Autodesk Inventor part; units mm, degrees
(part 3 of 7)
  arc A347 (-153.3618, 85.9364) -> (-153.2072, 86.2055) centre (-157.8537, 88.696) ccw projected
  arc A348 (-153.5785, 85.6068) -> (-153.3618, 85.9364) centre (-158.8215, 89.2905) ccw projected
  arc A349 (-153.872, 85.2164) -> (-153.5785, 85.6068) centre (-159.7867, 89.9687) ccw projected
  arc A350 (-154.2565, 85.3248) -> (-153.872, 85.2164) centre (-148.5, 105) ccw projected
  arc A351 (-154.3028, 85.8111) -> (-154.2565, 85.3248) centre (-146.7304, 86.2864) ccw projected
  arc A352 (-154.3154, 86.2053) -> (-154.3028, 85.8111) centre (-147.9076, 86.2125) ccw projected
  arc A353 (-154.3066, 86.5156) -> (-154.3154, 86.2053) centre (-149.0434, 86.2112) ccw projected
  arc A354 (-154.6673, 86.6328) -> (-154.3066, 86.5156) centre (-148.5, 105) ccw projected
  arc A355 (-154.8425, 86.3766) -> (-154.6673, 86.6328) centre (-159.1041, 89.4801) ccw projected
  arc A356 (-155.0844, 86.0651) -> (-154.8425, 86.3766) centre (-160.0222, 90.1488) ccw projected
  arc A357 (-155.4077, 85.6989) -> (-155.0844, 86.0651) centre (-160.9312, 90.9006) ccw projected
  arc A358 (-155.7825, 85.8371) -> (-155.4077, 85.6989) centre (-148.5, 105) ccw projected
  arc A359 (-155.7904, 86.3255) -> (-155.7825, 85.8371) centre (-148.2041, 86.2053) ccw projected
  arc A360 (-155.772, 86.7195) -> (-155.7904, 86.3255) centre (-149.3835, 86.224) ccw projected
  arc A361 (-155.7389, 87.0281) -> (-155.772, 86.7195) centre (-150.5159, 86.3118) ccw projected
  arc A362 (-156.0893, 87.1733) -> (-155.7389, 87.0281) centre (-148.5, 105) ccw projected
  arc A363 (-156.2842, 86.9316) -> (-156.0893, 87.1733) centre (-160.2891, 90.36) ccw projected
  arc A364 (-156.5497, 86.64) -> (-156.2842, 86.9316) centre (-161.1519, 91.0986) ccw projected
  arc A365 (-156.9007, 86.3003) -> (-156.5497, 86.64) centre (-161.9991, 91.9194) ccw projected
  arc A366 (-157.2635, 86.4676) -> (-156.9007, 86.3003) centre (-148.5, 105) ccw projected
  arc A367 (-157.2331, 86.9551) -> (-157.2635, 86.4676) centre (-149.6796, 86.24) ccw projected
  arc A368 (-157.1839, 87.3464) -> (-157.2331, 86.9551) centre (-150.8539, 86.3512) ccw projected
  arc A369 (-157.1267, 87.6515) -> (-157.1839, 87.3464) centre (-151.976, 86.5276) ccw projected
  arc A370 (-157.4646, 87.8237) -> (-157.1267, 87.6515) centre (-148.5, 105) ccw projected
  arc A371 (-157.6778, 87.5981) -> (-157.4646, 87.8237) centre (-161.4014, 91.3301) ccw projected
  arc A372 (-157.9654, 87.3282) -> (-157.6778, 87.5981) centre (-162.2036, 92.1341) ccw projected
  arc A373 (-158.342, 87.0171) -> (-157.9654, 87.3282) centre (-162.9838, 93.0188) ccw projected
  arc A374 (-158.6905, 87.2123) -> (-158.342, 87.0171) centre (-148.5, 105) ccw projected
  arc A375 (-158.622, 87.6959) -> (-158.6905, 87.2123) centre (-151.1478, 86.3904) ccw projected
  arc A376 (-158.5422, 88.0822) -> (-158.622, 87.6959) centre (-152.3099, 86.5933) ccw projected
  arc A377 (-158.4612, 88.3818) -> (-158.5422, 88.0822) centre (-153.4146, 86.8572) ccw projected
  arc A378 (-158.7846, 88.58) -> (-158.4612, 88.3818) centre (-148.5, 105) ccw projected
  arc A379 (-159.0148, 88.3718) -> (-158.7846, 88.58) centre (-162.4341, 92.3844) ccw projected
  arc A380 (-159.3227, 88.1253) -> (-159.0148, 88.3718) centre (-163.1708, 93.2489) ccw projected
  arc A381 (-159.7226, 87.8447) -> (-159.3227, 88.1253) centre (-163.8792, 94.1922) ccw projected
  arc A382 (-160.0547, 88.0666) -> (-159.7226, 87.8447) centre (-148.5, 105) ccw projected
  arc A383 (-159.9485, 88.5434) -> (-160.0547, 88.0666) centre (-152.5998, 86.6555) ccw projected
  arc A384 (-159.8386, 88.9222) -> (-159.9485, 88.5434) centre (-153.7423, 86.949) ccw projected
  arc A385 (-159.7344, 89.2146) -> (-159.8386, 88.9222) centre (-154.8229, 87.2988) ccw projected
  arc A386 (-160.0412, 89.4375) -> (-159.7344, 89.2146) centre (-148.5, 105) ccw projected
  arc A387 (-160.2871, 89.248) -> (-160.0412, 89.4375) centre (-163.381, 93.5166) ccw projected
  arc A388 (-160.6134, 89.0265) -> (-160.2871, 89.248) centre (-164.0476, 94.4362) ccw projected
  arc A389 (-161.034, 88.7781) -> (-160.6134, 89.0265) centre (-164.6798, 95.4321) ccw projected
  arc A390 (-161.3477, 89.0254) -> (-161.034, 88.7781) centre (-148.5, 105) ccw projected
  arc A391 (-161.2043, 89.4924) -> (-161.3477, 89.0254) centre (-154.0264, 87.0337) ccw projected
  arc A392 (-161.0651, 89.8614) -> (-161.2043, 89.4924) centre (-155.1424, 87.4159) ccw projected
  arc A393 (-160.9383, 90.1447) -> (-161.0651, 89.8614) centre (-156.1922, 87.8494) ccw projected
  arc A394 (-161.2266, 90.391) -> (-160.9383, 90.1447) centre (-148.5, 105) ccw projected
  arc A395 (-161.4866, 90.2214) -> (-161.2266, 90.391) centre (-164.2361, 94.7195) ccw projected
  arc A396 (-161.8293, 90.0261) -> (-161.4866, 90.2214) centre (-164.8285, 95.6886) ccw projected
  arc A397 (-162.2681, 89.8115) -> (-161.8293, 90.0261) centre (-165.3806, 96.7311) ccw projected
  arc A398 (-162.5614, 90.0827) -> (-162.2681, 89.8115) centre (-148.5, 105) ccw projected
  arc A399 (-162.3819, 90.537) -> (-162.5614, 90.0827) centre (-155.419, 87.5227) ccw projected
  arc A400 (-162.2141, 90.8939) -> (-162.3819, 90.537) centre (-156.5015, 87.9913) ccw projected
  arc A401 (-162.0655, 91.1664) -> (-162.2141, 90.8939) centre (-157.5141, 88.5058) ccw projected
  arc A402 (-162.3336, 91.4345) -> (-162.0655, 91.1664) centre (-148.5, 105) ccw projected
  arc A403 (-162.6061, 91.2859) -> (-162.3336, 91.4345) centre (-164.9942, 95.9859) ccw projected
  arc A404 (-162.963, 91.1181) -> (-162.6061, 91.2859) centre (-165.5087, 96.9985) ccw projected
  arc A405 (-163.4173, 90.9386) -> (-162.963, 91.1181) centre (-165.9773, 98.081) ccw projected
  arc A406 (-163.6885, 91.2319) -> (-163.4173, 90.9386) centre (-148.5, 105) ccw projected
  arc A407 (-163.4738, 91.6707) -> (-163.6885, 91.2319) centre (-156.7689, 88.1194) ccw projected
  arc A408 (-163.2786, 92.0134) -> (-163.4738, 91.6707) centre (-157.8114, 88.6715) ccw projected
  arc A409 (-163.109, 92.2734) -> (-163.2786, 92.0134) centre (-158.7805, 89.2639) ccw projected
  arc A410 (-163.3553, 92.5617) -> (-163.109, 92.2734) centre (-148.5, 105) ccw projected
  arc A411 (-163.6386, 92.4349) -> (-163.3553, 92.5617) centre (-165.6506, 97.3078) ccw projected
  arc A412 (-164.0076, 92.2957) -> (-163.6386, 92.4349) centre (-166.0841, 98.3576) ccw projected
  arc A413 (-164.4746, 92.1523) -> (-164.0076, 92.2957) centre (-166.4663, 99.4736) ccw projected
  arc A414 (-164.7219, 92.466) -> (-164.4746, 92.1523) centre (-148.5, 105) ccw projected
  arc A415 (-164.4735, 92.8866) -> (-164.7219, 92.466) centre (-158.0679, 88.8202) ccw projected
  arc A416 (-164.252, 93.2129) -> (-164.4735, 92.8866) centre (-159.0638, 89.4524) ccw projected
  arc A417 (-164.0625, 93.4588) -> (-164.252, 93.2129) centre (-159.9834, 90.119) ccw projected
  arc A418 (-164.2854, 93.7656) -> (-164.0625, 93.4588) centre (-148.5, 105) ccw projected
  arc A419 (-164.5778, 93.6614) -> (-164.2854, 93.7656) centre (-166.2012, 98.6771) ccw projected
  arc A420 (-164.9566, 93.5515) -> (-164.5778, 93.6614) centre (-166.551, 99.7577) ccw projected
  arc A421 (-165.4334, 93.4453) -> (-164.9566, 93.5515) centre (-166.8445, 100.9002) ccw projected
  arc A422 (-165.6553, 93.7774) -> (-165.4334, 93.4453) centre (-148.5, 105) ccw projected
  arc A423 (-165.3747, 94.1773) -> (-165.6553, 93.7774) centre (-159.3078, 89.6208) ccw projected
  arc A424 (-165.1282, 94.4852) -> (-165.3747, 94.1773) centre (-160.2511, 90.3292) ccw projected
  arc A425 (-164.92, 94.7154) -> (-165.1282, 94.4852) centre (-161.1156, 91.0659) ccw projected
  arc A426 (-165.1182, 95.0388) -> (-164.92, 94.7154) centre (-148.5, 105) ccw projected
  arc A427 (-165.4178, 94.9578) -> (-165.1182, 95.0388) centre (-166.6428, 100.0854) ccw projected
  arc A428 (-165.8041, 94.878) -> (-165.4178, 94.9578) centre (-166.9067, 101.1901) ccw projected
  arc A429 (-166.2877, 94.8095) -> (-165.8041, 94.878) centre (-167.1096, 102.3522) ccw projected
  arc A430 (-166.4829, 95.158) -> (-166.2877, 94.8095) centre (-148.5, 105) ccw projected
  arc A431 (-166.1718, 95.5346) -> (-166.4829, 95.158) centre (-160.4812, 90.5162) ccw projected
  arc A432 (-165.9019, 95.8222) -> (-166.1718, 95.5346) centre (-161.3659, 91.2964) ccw projected
  arc A433 (-165.6763, 96.0354) -> (-165.9019, 95.8222) centre (-162.1699, 92.0986) ccw projected
  arc A434 (-165.8485, 96.3733) -> (-165.6763, 96.0354) centre (-148.5, 105) ccw projected
  arc A435 (-166.1536, 96.3161) -> (-165.8485, 96.3733) centre (-166.9724, 101.524) ccw projected
  arc A436 (-166.5449, 96.2669) -> (-166.1536, 96.3161) centre (-167.1488, 102.6461) ccw projected
  arc A437 (-167.0324, 96.2365) -> (-166.5449, 96.2669) centre (-167.26, 103.8204) ccw projected
  arc A438 (-167.1997, 96.5993) -> (-167.0324, 96.2365) centre (-148.5, 105) ccw projected
  arc A439 (-166.86, 96.9503) -> (-167.1997, 96.5993) centre (-161.5806, 91.5009) ccw projected
  arc A440 (-166.5684, 97.2158) -> (-166.86, 96.9503) centre (-162.4014, 92.3481) ccw projected
  arc A441 (-166.3267, 97.4107) -> (-166.5684, 97.2158) centre (-163.14, 93.2109) ccw projected
  arc A442 (-166.4719, 97.7611) -> (-166.3267, 97.4107) centre (-148.5, 105) ccw projected
  arc A443 (-166.7805, 97.728) -> (-166.4719, 97.7611) centre (-167.1882, 102.9841) ccw projected
  arc A444 (-167.1745, 97.7096) -> (-166.7805, 97.728) centre (-167.276, 104.1165) ccw projected
  arc A445 (-167.6629, 97.7175) -> (-167.1745, 97.7096) centre (-167.2947, 105.2959) ccw projected
  arc A446 (-167.8011, 98.0923) -> (-167.6629, 97.7175) centre (-148.5, 105) ccw projected
  arc A447 (-167.4349, 98.4156) -> (-167.8011, 98.0923) centre (-162.5994, 92.5688) ccw projected
  arc A448 (-167.1234, 98.6575) -> (-167.4349, 98.4156) centre (-163.3512, 93.4778) ccw projected
  arc A449 (-166.8672, 98.8327) -> (-167.1234, 98.6575) centre (-164.0199, 94.3959) ccw projected
  arc A450 (-166.9844, 99.1934) -> (-166.8672, 98.8327) centre (-148.5, 105) ccw projected
  arc A451 (-167.2947, 99.1846) -> (-166.9844, 99.1934) centre (-167.2888, 104.4566) ccw projected
  arc A452 (-167.6889, 99.1972) -> (-167.2947, 99.1846) centre (-167.2875, 105.5924) ccw projected
  arc A453 (-168.1752, 99.2435) -> (-167.6889, 99.1972) centre (-167.2136, 106.7696) ccw projected
  arc A454 (-168.2836, 99.628) -> (-168.1752, 99.2435) centre (-148.5, 105) ccw projected
  arc A455 (-167.8932, 99.9215) -> (-168.2836, 99.628) centre (-163.5313, 93.7133) ccw projected
  arc A456 (-167.5636, 100.1382) -> (-167.8932, 99.9215) centre (-164.2095, 94.6785) ccw projected
  arc A457 (-167.2945, 100.2928) -> (-167.5636, 100.1382) centre (-164.804, 95.6463) ccw projected
  arc A458 (-167.383, 100.6616) -> (-167.2945, 100.2928) centre (-148.5, 105) ccw projected
  arc A459 (-167.693, 100.6772) -> (-167.383, 100.6616) centre (-167.2735, 105.9324) ccw projected
  arc A460 (-168.085, 100.7207) -> (-167.693, 100.6772) centre (-167.1831, 107.0646) ccw projected
  arc A461 (-168.5662, 100.8049) -> (-168.085, 100.7207) centre (-167.017, 108.2324) ccw projected
  arc A462 (-168.6441, 101.1967) -> (-168.5662, 100.8049) centre (-148.5, 105) ccw projected
  arc A463 (-168.2318, 101.4587) -> (-168.6441, 101.1967) centre (-164.3705, 94.9274) ccw projected
  arc A464 (-167.8863, 101.6489) -> (-168.2318, 101.4587) centre (-164.9708, 95.9429) ccw projected
  arc A465 (-167.6059, 101.7819) -> (-167.8863, 101.6489) centre (-165.4876, 96.9543) ccw projected
  arc A466 (-167.6652, 102.1565) -> (-167.6059, 101.7819) centre (-148.5, 105) ccw projected
  arc A467 (-167.973, 102.1964) -> (-167.6652, 102.1565) centre (-167.1425, 107.4025) ccw projected
  arc A468 (-168.3604, 102.2705) -> (-167.973, 102.1964) centre (-166.9635, 108.5241) ccw projected
  arc A469 (-168.8335, 102.3922) -> (-168.3604, 102.2705) centre (-166.7064, 109.6753) ccw projected
  arc A470 (-168.8804, 102.7889) -> (-168.8335, 102.3922) centre (-148.5, 105) ccw projected
  arc A471 (-168.4489, 103.0178) -> (-168.8804, 102.7889) centre (-165.1119, 96.2037) ccw projected
  arc A472 (-168.0895, 103.1803) -> (-168.4489, 103.0178) centre (-165.6307, 97.2631) ccw projected
  arc A473 (-167.7995, 103.2909) -> (-168.0895, 103.1803) centre (-166.0665, 98.3119) ccw projected
  arc A474 (-167.8292, 103.669) -> (-167.7995, 103.2909) centre (-148.5, 105) ccw projected
  arc A475 (-168.133, 103.7329) -> (-167.8292, 103.669) centre (-166.8965, 108.8577) ccw projected
  arc A476 (-168.5133, 103.8371) -> (-168.133, 103.7329) centre (-166.6301, 109.9618) ccw projected
  arc A477 (-168.9754, 103.9956) -> (-168.5133, 103.8371) centre (-166.2834, 111.0894) ccw projected
  arc A478 (-168.9911, 104.3948) -> (-168.9754, 103.9956) centre (-148.5, 105) ccw projected
  arc A479 (-168.5429, 104.5891) -> (-168.9911, 104.3948) centre (-165.7508, 97.5342) ccw projected
  arc A480 (-168.1719, 104.7229) -> (-168.5429, 104.5891) centre (-166.1849, 98.631) ccw projected
  arc A481 (-167.8741, 104.8104) -> (-168.1719, 104.7229) centre (-166.5371, 99.7108) ccw projected
  arc A482 (-167.8741, 105.1896) -> (-167.8741, 104.8104) centre (-148.5, 105) ccw projected
  arc A483 (-168.1719, 105.2771) -> (-167.8741, 105.1896) centre (-166.5371, 110.2892) ccw projected
  arc A484 (-168.5429, 105.4109) -> (-168.1719, 105.2771) centre (-166.1849, 111.369) ccw projected
  arc A485 (-168.9911, 105.6052) -> (-168.5429, 105.4109) centre (-165.7508, 112.4658) ccw projected
  arc A486 (-168.9754, 106.0044) -> (-168.9911, 105.6052) centre (-148.5, 105) ccw projected
  arc A487 (-168.5133, 106.1629) -> (-168.9754, 106.0044) centre (-166.2834, 98.9106) ccw projected
  arc A488 (-168.133, 106.2671) -> (-168.5133, 106.1629) centre (-166.6301, 100.0382) ccw projected
  arc A489 (-167.8292, 106.331) -> (-168.133, 106.2671) centre (-166.8965, 101.1423) ccw projected
  arc A490 (-167.7995, 106.7091) -> (-167.8292, 106.331) centre (-148.5, 105) ccw projected
  arc A491 (-168.0895, 106.8197) -> (-167.7995, 106.7091) centre (-166.0665, 111.6881) ccw projected
  arc A492 (-168.4489, 106.9822) -> (-168.0895, 106.8197) centre (-165.6307, 112.7369) ccw projected
  arc A493 (-168.8804, 107.2111) -> (-168.4489, 106.9822) centre (-165.1119, 113.7963) ccw projected
  arc A494 (-168.8335, 107.6078) -> (-168.8804, 107.2111) centre (-148.5, 105) ccw projected
  arc A495 (-168.3604, 107.7295) -> (-168.8335, 107.6078) centre (-166.7064, 100.3247) ccw projected
  arc A496 (-167.973, 107.8036) -> (-168.3604, 107.7295) centre (-166.9635, 101.4759) ccw projected
  arc A497 (-167.6652, 107.8435) -> (-167.973, 107.8036) centre (-167.1425, 102.5975) ccw projected
  arc A498 (-167.6059, 108.2181) -> (-167.6652, 107.8435) centre (-148.5, 105) ccw projected
  arc A499 (-167.8863, 108.3511) -> (-167.6059, 108.2181) centre (-165.4876, 113.0457) ccw projected
  arc A500 (-168.2318, 108.5413) -> (-167.8863, 108.3511) centre (-164.9708, 114.0571) ccw projected
  arc A501 (-168.6441, 108.8033) -> (-168.2318, 108.5413) centre (-164.3705, 115.0726) ccw projected
  arc A502 (-168.5662, 109.1951) -> (-168.6441, 108.8033) centre (-148.5, 105) ccw projected
  arc A503 (-168.085, 109.2793) -> (-168.5662, 109.1951) centre (-167.017, 101.7676) ccw projected
  arc A504 (-167.693, 109.3228) -> (-168.085, 109.2793) centre (-167.1831, 102.9354) ccw projected
  arc A505 (-167.383, 109.3384) -> (-167.693, 109.3228) centre (-167.2735, 104.0676) ccw projected
  arc A506 (-167.2945, 109.7072) -> (-167.383, 109.3384) centre (-148.5, 105) ccw projected
  arc A507 (-167.5636, 109.8618) -> (-167.2945, 109.7072) centre (-164.804, 114.3537) ccw projected
  arc A508 (-167.8932, 110.0785) -> (-167.5636, 109.8618) centre (-164.2095, 115.3215) ccw projected
  arc A509 (-168.2836, 110.372) -> (-167.8932, 110.0785) centre (-163.5313, 116.2867) ccw projected
  arc A510 (-168.1752, 110.7565) -> (-168.2836, 110.372) centre (-148.5, 105) ccw projected
  arc A511 (-167.6889, 110.8028) -> (-168.1752, 110.7565) centre (-167.2136, 103.2304) ccw projected
  arc A512 (-167.2947, 110.8154) -> (-167.6889, 110.8028) centre (-167.2875, 104.4076) ccw projected
  arc A513 (-166.9844, 110.8066) -> (-167.2947, 110.8154) centre (-167.2888, 105.5434) ccw projected
  arc A514 (-166.8672, 111.1673) -> (-166.9844, 110.8066) centre (-148.5, 105) ccw projected
  arc A515 (-167.1234, 111.3425) -> (-166.8672, 111.1673) centre (-164.0199, 115.6041) ccw projected
  arc A516 (-167.4349, 111.5844) -> (-167.1234, 111.3425) centre (-163.3512, 116.5222) ccw projected
  arc A517 (-167.8011, 111.9077) -> (-167.4349, 111.5844) centre (-162.5994, 117.4312) ccw projected
  arc A518 (-167.6629, 112.2825) -> (-167.8011, 111.9077) centre (-148.5, 105) ccw projected
  arc A519 (-167.1745, 112.2904) -> (-167.6629, 112.2825) centre (-167.2947, 104.7041) ccw projected
  arc A520 (-166.7805, 112.272) -> (-167.1745, 112.2904) centre (-167.276, 105.8835) ccw projected
  arc A521 (-166.4719, 112.2389) -> (-166.7805, 112.272) centre (-167.1882, 107.0159) ccw projected
  arc A522 (-166.3267, 112.5893) -> (-166.4719, 112.2389) centre (-148.5, 105) ccw projected
  arc A523 (-166.5684, 112.7842) -> (-166.3267, 112.5893) centre (-163.14, 116.7891) ccw projected
  arc A524 (-166.86, 113.0497) -> (-166.5684, 112.7842) centre (-162.4014, 117.6519) ccw projected
  arc A525 (-167.1997, 113.4007) -> (-166.86, 113.0497) centre (-161.5806, 118.4991) ccw projected
  arc A526 (-167.0324, 113.7635) -> (-167.1997, 113.4007) centre (-148.5, 105) ccw projected
  arc A527 (-166.5449, 113.7331) -> (-167.0324, 113.7635) centre (-167.26, 106.1796) ccw projected
  arc A528 (-166.1536, 113.6839) -> (-166.5449, 113.7331) centre (-167.1488, 107.3539) ccw projected
  arc A529 (-165.8485, 113.6267) -> (-166.1536, 113.6839) centre (-166.9724, 108.476) ccw projected
  arc A530 (-165.6763, 113.9646) -> (-165.8485, 113.6267) centre (-148.5, 105) ccw projected
  arc A531 (-165.9019, 114.1778) -> (-165.6763, 113.9646) centre (-162.1699, 117.9014) ccw projected
  arc A532 (-166.1718, 114.4654) -> (-165.9019, 114.1778) centre (-161.3659, 118.7036) ccw projected
  arc A533 (-166.4829, 114.842) -> (-166.1718, 114.4654) centre (-160.4812, 119.4838) ccw projected
  arc A534 (-166.2877, 115.1905) -> (-166.4829, 114.842) centre (-148.5, 105) ccw projected
  arc A535 (-165.8041, 115.122) -> (-166.2877, 115.1905) centre (-167.1096, 107.6478) ccw projected
  arc A536 (-165.4178, 115.0422) -> (-165.8041, 115.122) centre (-166.9067, 108.8099) ccw projected
  arc A537 (-165.1182, 114.9612) -> (-165.4178, 115.0422) centre (-166.6428, 109.9146) ccw projected
  arc A538 (-164.92, 115.2846) -> (-165.1182, 114.9612) centre (-148.5, 105) ccw projected
  arc A539 (-165.1282, 115.5148) -> (-164.92, 115.2846) centre (-161.1156, 118.9341) ccw projected
  arc A540 (-165.3747, 115.8227) -> (-165.1282, 115.5148) centre (-160.2511, 119.6708) ccw projected
  arc A541 (-165.6553, 116.2226) -> (-165.3747, 115.8227) centre (-159.3078, 120.3792) ccw projected
  arc A542 (-165.4334, 116.5547) -> (-165.6553, 116.2226) centre (-148.5, 105) ccw projected
  arc A543 (-164.9566, 116.4485) -> (-165.4334, 116.5547) centre (-166.8445, 109.0998) ccw projected
  arc A544 (-164.5778, 116.3386) -> (-164.9566, 116.4485) centre (-166.551, 110.2423) ccw projected
  arc A545 (-164.2854, 116.2344) -> (-164.5778, 116.3386) centre (-166.2012, 111.3229) ccw projected
  arc A546 (-164.0625, 116.5412) -> (-164.2854, 116.2344) centre (-148.5, 105) ccw projected
  arc A547 (-164.252, 116.7871) -> (-164.0625, 116.5412) centre (-159.9834, 119.881) ccw projected
  arc A548 (-164.4735, 117.1134) -> (-164.252, 116.7871) centre (-159.0638, 120.5476) ccw projected
  arc A549 (-164.7219, 117.534) -> (-164.4735, 117.1134) centre (-158.0679, 121.1798) ccw projected
  arc A550 (-164.4746, 117.8477) -> (-164.7219, 117.534) centre (-148.5, 105) ccw projected
  arc A551 (-164.0076, 117.7043) -> (-164.4746, 117.8477) centre (-166.4663, 110.5264) ccw projected
  arc A552 (-163.6386, 117.5651) -> (-164.0076, 117.7043) centre (-166.0841, 111.6424) ccw projected
  arc A553 (-163.3553, 117.4383) -> (-163.6386, 117.5651) centre (-165.6506, 112.6922) ccw projected
  arc A554 (-163.109, 117.7266) -> (-163.3553, 117.4383) centre (-148.5, 105) ccw projected
  arc A555 (-163.2786, 117.9866) -> (-163.109, 117.7266) centre (-158.7805, 120.7361) ccw projected
  arc A556 (-163.4738, 118.3293) -> (-163.2786, 117.9866) centre (-157.8114, 121.3285) ccw projected
  arc A557 (-163.6885, 118.7681) -> (-163.4738, 118.3293) centre (-156.7689, 121.8806) ccw projected
  arc A558 (-163.4173, 119.0614) -> (-163.6885, 118.7681) centre (-148.5, 105) ccw projected
  arc A559 (-162.963, 118.8819) -> (-163.4173, 119.0614) centre (-165.9773, 111.919) ccw projected
  arc A560 (-162.6061, 118.7141) -> (-162.963, 118.8819) centre (-165.5087, 113.0015) ccw projected
  arc A561 (-162.3336, 118.5655) -> (-162.6061, 118.7141) centre (-164.9942, 114.0141) ccw projected
  arc A562 (-162.0655, 118.8336) -> (-162.3336, 118.5655) centre (-148.5, 105) ccw projected
  arc A563 (-162.2141, 119.1061) -> (-162.0655, 118.8336) centre (-157.5141, 121.4942) ccw projected
  arc A564 (-162.3819, 119.463) -> (-162.2141, 119.1061) centre (-156.5015, 122.0087) ccw projected
  arc A565 (-162.5614, 119.9173) -> (-162.3819, 119.463) centre (-155.419, 122.4773) ccw projected
  arc A566 (-162.2681, 120.1885) -> (-162.5614, 119.9173) centre (-148.5, 105) ccw projected
  arc A567 (-161.8293, 119.9739) -> (-162.2681, 120.1885) centre (-165.3806, 113.2689) ccw projected
  arc A568 (-161.4866, 119.7786) -> (-161.8293, 119.9739) centre (-164.8285, 114.3114) ccw projected
  arc A569 (-161.2266, 119.609) -> (-161.4866, 119.7786) centre (-164.2361, 115.2805) ccw projected
  arc A570 (-160.9383, 119.8553) -> (-161.2266, 119.609) centre (-148.5, 105) ccw projected
  arc A571 (-161.0651, 120.1386) -> (-160.9383, 119.8553) centre (-156.1922, 122.1506) ccw projected
  arc A572 (-161.2043, 120.5076) -> (-161.0651, 120.1386) centre (-155.1424, 122.5841) ccw projected
  arc A573 (-161.3477, 120.9746) -> (-161.2043, 120.5076) centre (-154.0264, 122.9663) ccw projected
  arc A574 (-161.034, 121.2219) -> (-161.3477, 120.9746) centre (-148.5, 105) ccw projected
  arc A575 (-160.6134, 120.9735) -> (-161.034, 121.2219) centre (-164.6798, 114.5679) ccw projected
  arc A576 (-160.2871, 120.752) -> (-160.6134, 120.9735) centre (-164.0476, 115.5638) ccw projected
  arc A577 (-160.0412, 120.5625) -> (-160.2871, 120.752) centre (-163.381, 116.4834) ccw projected
  arc A578 (-159.7344, 120.7854) -> (-160.0412, 120.5625) centre (-148.5, 105) ccw projected
  arc A579 (-159.8386, 121.0778) -> (-159.7344, 120.7854) centre (-154.8229, 122.7012) ccw projected
  arc A580 (-159.9485, 121.4566) -> (-159.8386, 121.0778) centre (-153.7423, 123.051) ccw projected
  arc A581 (-160.0547, 121.9334) -> (-159.9485, 121.4566) centre (-152.5998, 123.3445) ccw projected
  arc A582 (-159.7226, 122.1553) -> (-160.0547, 121.9334) centre (-148.5, 105) ccw projected
  arc A583 (-159.3227, 121.8747) -> (-159.7226, 122.1553) centre (-163.8792, 115.8078) ccw projected
  arc A584 (-159.0148, 121.6282) -> (-159.3227, 121.8747) centre (-163.1708, 116.7511) ccw projected
  arc A585 (-158.7846, 121.42) -> (-159.0148, 121.6282) centre (-162.4341, 117.6156) ccw projected
  arc A586 (-158.4612, 121.6182) -> (-158.7846, 121.42) centre (-148.5, 105) ccw projected
  arc A587 (-158.5422, 121.9178) -> (-158.4612, 121.6182) centre (-153.4146, 123.1428) ccw projected
  arc A588 (-158.622, 122.3041) -> (-158.5422, 121.9178) centre (-152.3099, 123.4067) ccw projected
  arc A589 (-158.6905, 122.7877) -> (-158.622, 122.3041) centre (-151.1478, 123.6096) ccw projected
  arc A590 (-158.342, 122.9829) -> (-158.6905, 122.7877) centre (-148.5, 105) ccw projected
  arc A591 (-157.9654, 122.6718) -> (-158.342, 122.9829) centre (-162.9838, 116.9812) ccw projected
  arc A592 (-157.6778, 122.4019) -> (-157.9654, 122.6718) centre (-162.2036, 117.8659) ccw projected
  arc A593 (-157.4646, 122.1763) -> (-157.6778, 122.4019) centre (-161.4014, 118.6699) ccw projected
  arc A594 (-157.1267, 122.3485) -> (-157.4646, 122.1763) centre (-148.5, 105) ccw projected
  arc A595 (-157.1839, 122.6536) -> (-157.1267, 122.3485) centre (-151.976, 123.4724) ccw projected
  arc A596 (-157.2331, 123.0449) -> (-157.1839, 122.6536) centre (-150.8539, 123.6488) ccw projected
  arc A597 (-157.2635, 123.5324) -> (-157.2331, 123.0449) centre (-149.6796, 123.76) ccw projected
  arc A598 (-156.9007, 123.6997) -> (-157.2635, 123.5324) centre (-148.5, 105) ccw projected
  arc A599 (-156.5497, 123.36) -> (-156.9007, 123.6997) centre (-161.9991, 118.0806) ccw projected
  arc A600 (-156.2842, 123.0684) -> (-156.5497, 123.36) centre (-161.1519, 118.9014) ccw projected
  arc A601 (-156.0893, 122.8267) -> (-156.2842, 123.0684) centre (-160.2891, 119.64) ccw projected
  arc A602 (-155.7389, 122.9719) -> (-156.0893, 122.8267) centre (-148.5, 105) ccw projected
  arc A603 (-155.772, 123.2805) -> (-155.7389, 122.9719) centre (-150.5159, 123.6882) ccw projected
  arc A604 (-155.7904, 123.6745) -> (-155.772, 123.2805) centre (-149.3835, 123.776) ccw projected
  arc A605 (-155.7825, 124.1629) -> (-155.7904, 123.6745) centre (-148.2041, 123.7947) ccw projected
  arc A606 (-155.4077, 124.3011) -> (-155.7825, 124.1629) centre (-148.5, 105) ccw projected
  arc A607 (-155.0844, 123.9349) -> (-155.4077, 124.3011) centre (-160.9312, 119.0994) ccw projected
  arc A608 (-154.8425, 123.6234) -> (-155.0844, 123.9349) centre (-160.0222, 119.8512) ccw projected
  arc A609 (-154.6673, 123.3672) -> (-154.8425, 123.6234) centre (-159.1041, 120.5199) ccw projected
  arc A610 (-154.3066, 123.4844) -> (-154.6673, 123.3672) centre (-148.5, 105) ccw projected
  arc A611 (-154.3154, 123.7947) -> (-154.3066, 123.4844) centre (-149.0434, 123.7888) ccw projected
  arc A612 (-154.3028, 124.1889) -> (-154.3154, 123.7947) centre (-147.9076, 123.7875) ccw projected
  arc A613 (-154.2565, 124.6752) -> (-154.3028, 124.1889) centre (-146.7304, 123.7136) ccw projected
  arc A614 (-153.872, 124.7836) -> (-154.2565, 124.6752) centre (-148.5, 105) ccw projected
  arc A615 (-153.5785, 124.3932) -> (-153.872, 124.7836) centre (-159.7867, 120.0313) ccw projected
  arc A616 (-153.3618, 124.0636) -> (-153.5785, 124.3932) centre (-158.8215, 120.7095) ccw projected
  arc A617 (-153.2072, 123.7945) -> (-153.3618, 124.0636) centre (-157.8537, 121.304) ccw projected
  arc A618 (-152.8384, 123.883) -> (-153.2072, 123.7945) centre (-148.5, 105) ccw projected
  arc A619 (-152.8228, 124.193) -> (-152.8384, 123.883) centre (-147.5676, 123.7735) ccw projected
  arc A620 (-152.7793, 124.585) -> (-152.8228, 124.193) centre (-146.4354, 123.6831) ccw projected
  arc A621 (-152.6951, 125.0662) -> (-152.7793, 124.585) centre (-145.2676, 123.517) ccw projected
  arc A622 (-152.3033, 125.1441) -> (-152.6951, 125.0662) centre (-148.5, 105) ccw projected
  arc A623 (-152.0413, 124.7318) -> (-152.3033, 125.1441) centre (-158.5726, 120.8705) ccw projected
  arc A624 (-151.8511, 124.3863) -> (-152.0413, 124.7318) centre (-157.5571, 121.4708) ccw projected
  arc A625 (-151.7181, 124.1059) -> (-151.8511, 124.3863) centre (-156.5457, 121.9876) ccw projected
  arc A626 (-151.3435, 124.1652) -> (-151.7181, 124.1059) centre (-148.5, 105) ccw projected
  arc A627 (-151.3036, 124.473) -> (-151.3435, 124.1652) centre (-146.0975, 123.6425) ccw projected
  arc A628 (-151.2295, 124.8604) -> (-151.3036, 124.473) centre (-144.9759, 123.4635) ccw projected
  arc A629 (-151.1078, 125.3335) -> (-151.2295, 124.8604) centre (-143.8247, 123.2064) ccw projected
  arc A630 (-150.7111, 125.3804) -> (-151.1078, 125.3335) centre (-148.5, 105) ccw projected
  arc A631 (-150.4822, 124.9489) -> (-150.7111, 125.3804) centre (-157.2963, 121.6119) ccw projected
  arc A632 (-150.3197, 124.5895) -> (-150.4822, 124.9489) centre (-156.2369, 122.1307) ccw projected
  arc A633 (-150.2091, 124.2995) -> (-150.3197, 124.5895) centre (-155.1881, 122.5665) ccw projected
  arc A634 (-149.831, 124.3292) -> (-150.2091, 124.2995) centre (-148.5, 105) ccw projected
  arc A635 (-149.7671, 124.633) -> (-149.831, 124.3292) centre (-144.6423, 123.3965) ccw projected
  arc A636 (-149.6629, 125.0133) -> (-149.7671, 124.633) centre (-143.5382, 123.1301) ccw projected
  arc A637 (-149.5044, 125.4754) -> (-149.6629, 125.0133) centre (-142.4106, 122.7834) ccw projected
  arc A638 (-149.1052, 125.4911) -> (-149.5044, 125.4754) centre (-148.5, 105) ccw projected
  arc A639 (-148.9109, 125.0429) -> (-149.1052, 125.4911) centre (-155.9658, 122.2508) ccw projected
  circle A640 centre (-148.5, 105) radius 6
  circle A641 centre (-148.5, 105) radius 18.25
  point P0 (0, 0)
  dimension "d11" = 12
  dimension "d12" = 36.5
  constraints: 2 centre point, 2 coincident
  measures "d11" diameter of A640
  measures "d12" diameter of A641
extrude "押し出し3" cut sketch "スケッチ3" against normal blind 0.75 contours A641
sketch "スケッチ4" plane through (0, 0, 3) normal (0, 0, 1) x (1, 0, 0)
  arc A0 (148.9109, 125.0429) -> (148.7771, 124.6719) centre (154.869, 122.6849) ccw projected
  arc A1 (149.1052, 125.4911) -> (148.9109, 125.0429) centre (155.9658, 122.2508) ccw projected
  arc A2 (149.5044, 125.4754) -> (149.1052, 125.4911) centre (148.5, 105) ccw projected
  arc A3 (149.6629, 125.0133) -> (149.5044, 125.4754) centre (142.4106, 122.7834) ccw projected
  arc A4 (149.7671, 124.633) -> (149.6629, 125.0133) centre (143.5382, 123.1301) ccw projected
  arc A5 (149.831, 124.3292) -> (149.7671, 124.633) centre (144.6423, 123.3965) ccw projected
  arc A6 (150.2091, 124.2995) -> (149.831, 124.3292) centre (148.5, 105) ccw projected
  arc A7 (150.3197, 124.5895) -> (150.2091, 124.2995) centre (155.1881, 122.5665) ccw projected
  arc A8 (150.4822, 124.9489) -> (150.3197, 124.5895) centre (156.2369, 122.1307) ccw projected
  arc A9 (150.7111, 125.3804) -> (150.4822, 124.9489) centre (157.2963, 121.6119) ccw projected
  arc A10 (151.1078, 125.3335) -> (150.7111, 125.3804) centre (148.5, 105) ccw projected
  arc A11 (151.2295, 124.8604) -> (151.1078, 125.3335) centre (143.8247, 123.2064) ccw projected
  arc A12 (151.3036, 124.473) -> (151.2295, 124.8604) centre (144.9759, 123.4635) ccw projected
  arc A13 (151.3435, 124.1652) -> (151.3036, 124.473) centre (146.0975, 123.6425) ccw projected
  arc A14 (151.7181, 124.1059) -> (151.3435, 124.1652) centre (148.5, 105) ccw projected
  arc A15 (151.8511, 124.3863) -> (151.7181, 124.1059) centre (156.5457, 121.9876) ccw projected
  arc A16 (152.0413, 124.7318) -> (151.8511, 124.3863) centre (157.5571, 121.4708) ccw projected
  arc A17 (152.3033, 125.1441) -> (152.0413, 124.7318) centre (158.5726, 120.8705) ccw projected
  arc A18 (152.6951, 125.0662) -> (152.3033, 125.1441) centre (148.5, 105) ccw projected
  arc A19 (152.7793, 124.585) -> (152.6951, 125.0662) centre (145.2676, 123.517) ccw projected
  arc A20 (152.8228, 124.193) -> (152.7793, 124.585) centre (146.4354, 123.6831) ccw projected
  arc A21 (152.8384, 123.883) -> (152.8228, 124.193) centre (147.5676, 123.7735) ccw projected
  arc A22 (153.2072, 123.7945) -> (152.8384, 123.883) centre (148.5, 105) ccw projected
  arc A23 (153.3618, 124.0636) -> (153.2072, 123.7945) centre (157.8537, 121.304) ccw projected
  arc A24 (153.5785, 124.3932) -> (153.3618, 124.0636) centre (158.8215, 120.7095) ccw projected
  arc A25 (153.872, 124.7836) -> (153.5785, 124.3932) centre (159.7867, 120.0313) ccw projected
  arc A26 (154.2565, 124.6752) -> (153.872, 124.7836) centre (148.5, 105) ccw projected
  arc A27 (154.3028, 124.1889) -> (154.2565, 124.6752) centre (146.7304, 123.7136) ccw projected
  arc A28 (154.3154, 123.7947) -> (154.3028, 124.1889) centre (147.9076, 123.7875) ccw projected
  arc A29 (154.3066, 123.4844) -> (154.3154, 123.7947) centre (149.0434, 123.7888) ccw projected
  arc A30 (154.6673, 123.3672) -> (154.3066, 123.4844) centre (148.5, 105) ccw projected
  arc A31 (154.8425, 123.6234) -> (154.6673, 123.3672) centre (159.1041, 120.5199) ccw projected
  arc A32 (155.0844, 123.9349) -> (154.8425, 123.6234) centre (160.0222, 119.8512) ccw projected
  arc A33 (155.4077, 124.3011) -> (155.0844, 123.9349) centre (160.9312, 119.0994) ccw projected
  arc A34 (155.7825, 124.1629) -> (155.4077, 124.3011) centre (148.5, 105) ccw projected
  arc A35 (155.7904, 123.6745) -> (155.7825, 124.1629) centre (148.2041, 123.7947) ccw projected
  arc A36 (155.772, 123.2805) -> (155.7904, 123.6745) centre (149.3835, 123.776) ccw projected
  arc A37 (155.7389, 122.9719) -> (155.772, 123.2805) centre (150.5159, 123.6882) ccw projected
  arc A38 (156.0893, 122.8267) -> (155.7389, 122.9719) centre (148.5, 105) ccw projected
  arc A39 (156.2842, 123.0684) -> (156.0893, 122.8267) centre (160.2891, 119.64) ccw projected
  arc A40 (156.5497, 123.36) -> (156.2842, 123.0684) centre (161.1519, 118.9014) ccw projected
  arc A41 (156.9007, 123.6997) -> (156.5497, 123.36) centre (161.9991, 118.0806) ccw projected
  arc A42 (157.2635, 123.5324) -> (156.9007, 123.6997) centre (148.5, 105) ccw projected
  arc A43 (157.2331, 123.0449) -> (157.2635, 123.5324) centre (149.6796, 123.76) ccw projected
  arc A44 (157.1839, 122.6536) -> (157.2331, 123.0449) centre (150.8539, 123.6488) ccw projected
  arc A45 (157.1267, 122.3485) -> (157.1839, 122.6536) centre (151.976, 123.4724) ccw projected
  arc A46 (157.4646, 122.1763) -> (157.1267, 122.3485) centre (148.5, 105) ccw projected
  arc A47 (157.6778, 122.4019) -> (157.4646, 122.1763) centre (161.4014, 118.6699) ccw projected
  arc A48 (157.9654, 122.6718) -> (157.6778, 122.4019) centre (162.2036, 117.8659) ccw projected
  arc A49 (158.342, 122.9829) -> (157.9654, 122.6718) centre (162.9838, 116.9812) ccw projected
  arc A50 (158.6905, 122.7877) -> (158.342, 122.9829) centre (148.5, 105) ccw projected
  arc A51 (158.622, 122.3041) -> (158.6905, 122.7877) centre (151.1478, 123.6096) ccw projected
  arc A52 (158.5422, 121.9178) -> (158.622, 122.3041) centre (152.3099, 123.4067) ccw projected
  arc A53 (158.4612, 121.6182) -> (158.5422, 121.9178) centre (153.4146, 123.1428) ccw projected
  arc A54 (158.7846, 121.42) -> (158.4612, 121.6182) centre (148.5, 105) ccw projected
  arc A55 (159.0148, 121.6282) -> (158.7846, 121.42) centre (162.4341, 117.6156) ccw projected
  arc A56 (159.3227, 121.8747) -> (159.0148, 121.6282) centre (163.1708, 116.7511) ccw projected
  arc A57 (159.7226, 122.1553) -> (159.3227, 121.8747) centre (163.8792, 115.8078) ccw projected
  arc A58 (160.0547, 121.9334) -> (159.7226, 122.1553) centre (148.5, 105) ccw projected
  arc A59 (159.9485, 121.4566) -> (160.0547, 121.9334) centre (152.5998, 123.3445) ccw projected
  arc A60 (159.8386, 121.0778) -> (159.9485, 121.4566) centre (153.7423, 123.051) ccw projected
  arc A61 (159.7344, 120.7854) -> (159.8386, 121.0778) centre (154.8229, 122.7012) ccw projected
  arc A62 (160.0412, 120.5625) -> (159.7344, 120.7854) centre (148.5, 105) ccw projected
  arc A63 (160.2871, 120.752) -> (160.0412, 120.5625) centre (163.381, 116.4834) ccw projected
  arc A64 (160.6134, 120.9735) -> (160.2871, 120.752) centre (164.0476, 115.5638) ccw projected
  arc A65 (161.034, 121.2219) -> (160.6134, 120.9735) centre (164.6798, 114.5679) ccw projected
  arc A66 (161.3477, 120.9746) -> (161.034, 121.2219) centre (148.5, 105) ccw projected
  arc A67 (161.2043, 120.5076) -> (161.3477, 120.9746) centre (154.0264, 122.9663) ccw projected
  arc A68 (161.0651, 120.1386) -> (161.2043, 120.5076) centre (155.1424, 122.5841) ccw projected
  arc A69 (160.9383, 119.8553) -> (161.0651, 120.1386) centre (156.1922, 122.1506) ccw projected
  arc A70 (161.2266, 119.609) -> (160.9383, 119.8553) centre (148.5, 105) ccw projected
  arc A71 (161.4866, 119.7786) -> (161.2266, 119.609) centre (164.2361, 115.2805) ccw projected
  arc A72 (161.8293, 119.9739) -> (161.4866, 119.7786) centre (164.8285, 114.3114) ccw projected
  arc A73 (162.2681, 120.1885) -> (161.8293, 119.9739) centre (165.3806, 113.2689) ccw projected
  arc A74 (162.5614, 119.9173) -> (162.2681, 120.1885) centre (148.5, 105) ccw projected
  arc A75 (162.3819, 119.463) -> (162.5614, 119.9173) centre (155.419, 122.4773) ccw projected
  arc A76 (162.2141, 119.1061) -> (162.3819, 119.463) centre (156.5015, 122.0087) ccw projected
  arc A77 (162.0655, 118.8336) -> (162.2141, 119.1061) centre (157.5141, 121.4942) ccw projected
  arc A78 (162.3336, 118.5655) -> (162.0655, 118.8336) centre (148.5, 105) ccw projected
  arc A79 (162.6061, 118.7141) -> (162.3336, 118.5655) centre (164.9942, 114.0141) ccw projected
  arc A80 (162.963, 118.8819) -> (162.6061, 118.7141) centre (165.5087, 113.0015) ccw projected
  arc A81 (163.4173, 119.0614) -> (162.963, 118.8819) centre (165.9773, 111.919) ccw projected
  arc A82 (163.6885, 118.7681) -> (163.4173, 119.0614) centre (148.5, 105) ccw projected
  arc A83 (163.4738, 118.3293) -> (163.6885, 118.7681) centre (156.7689, 121.8806) ccw projected
  arc A84 (163.2786, 117.9866) -> (163.4738, 118.3293) centre (157.8114, 121.3285) ccw projected
  arc A85 (163.109, 117.7266) -> (163.2786, 117.9866) centre (158.7805, 120.7361) ccw projected
  arc A86 (163.3553, 117.4383) -> (163.109, 117.7266) centre (148.5, 105) ccw projected
  arc A87 (163.6386, 117.5651) -> (163.3553, 117.4383) centre (165.6506, 112.6922) ccw projected
  arc A88 (164.0076, 117.7043) -> (163.6386, 117.5651) centre (166.0841, 111.6424) ccw projected
  arc A89 (164.4746, 117.8477) -> (164.0076, 117.7043) centre (166.4663, 110.5264) ccw projected
  arc A90 (164.7219, 117.534) -> (164.4746, 117.8477) centre (148.5, 105) ccw projected
  arc A91 (164.4735, 117.1134) -> (164.7219, 117.534) centre (158.0679, 121.1798) ccw projected
  arc A92 (164.252, 116.7871) -> (164.4735, 117.1134) centre (159.0638, 120.5476) ccw projected
  arc A93 (164.0625, 116.5412) -> (164.252, 116.7871) centre (159.9834, 119.881) ccw projected
  arc A94 (164.2854, 116.2344) -> (164.0625, 116.5412) centre (148.5, 105) ccw projected
  arc A95 (164.5778, 116.3386) -> (164.2854, 116.2344) centre (166.2012, 111.3229) ccw projected
  arc A96 (164.9566, 116.4485) -> (164.5778, 116.3386) centre (166.551, 110.2423) ccw projected
  arc A97 (165.4334, 116.5547) -> (164.9566, 116.4485) centre (166.8445, 109.0998) ccw projected
  arc A98 (165.6553, 116.2226) -> (165.4334, 116.5547) centre (148.5, 105) ccw projected
  arc A99 (165.3747, 115.8227) -> (165.6553, 116.2226) centre (159.3078, 120.3792) ccw projected
  arc A100 (165.1282, 115.5148) -> (165.3747, 115.8227) centre (160.2511, 119.6708) ccw projected
  arc A101 (164.92, 115.2846) -> (165.1282, 115.5148) centre (161.1156, 118.9341) ccw projected
  arc A102 (165.1182, 114.9612) -> (164.92, 115.2846) centre (148.5, 105) ccw projected
  arc A103 (165.4178, 115.0422) -> (165.1182, 114.9612) centre (166.6428, 109.9146) ccw projected
  arc A104 (165.8041, 115.122) -> (165.4178, 115.0422) centre (166.9067, 108.8099) ccw projected
  arc A105 (166.2877, 115.1905) -> (165.8041, 115.122) centre (167.1096, 107.6478) ccw projected
  arc A106 (166.4829, 114.842) -> (166.2877, 115.1905) centre (148.5, 105) ccw projected
  arc A107 (166.1718, 114.4654) -> (166.4829, 114.842) centre (160.4812, 119.4838) ccw projected
  arc A108 (165.9019, 114.1778) -> (166.1718, 114.4654) centre (161.3659, 118.7036) ccw projected
  arc A109 (165.6763, 113.9646) -> (165.9019, 114.1778) centre (162.1699, 117.9014) ccw projected
  arc A110 (165.8485, 113.6267) -> (165.6763, 113.9646) centre (148.5, 105) ccw projected
  arc A111 (166.1536, 113.6839) -> (165.8485, 113.6267) centre (166.9724, 108.476) ccw projected
  arc A112 (166.5449, 113.7331) -> (166.1536, 113.6839) centre (167.1488, 107.3539) ccw projected
  arc A113 (167.0324, 113.7635) -> (166.5449, 113.7331) centre (167.26, 106.1796) ccw projected
  arc A114 (167.1997, 113.4007) -> (167.0324, 113.7635) centre (148.5, 105) ccw projected
  arc A115 (166.86, 113.0497) -> (167.1997, 113.4007) centre (161.5806, 118.4991) ccw projected
  arc A116 (166.5684, 112.7842) -> (166.86, 113.0497) centre (162.4014, 117.6519) ccw projected
  arc A117 (166.3267, 112.5893) -> (166.5684, 112.7842) centre (163.14, 116.7891) ccw projected
  arc A118 (166.4719, 112.2389) -> (166.3267, 112.5893) centre (148.5, 105) ccw projected
  arc A119 (166.7805, 112.272) -> (166.4719, 112.2389) centre (167.1882, 107.0159) ccw projected
  arc A120 (167.1745, 112.2904) -> (166.7805, 112.272) centre (167.276, 105.8835) ccw projected
  arc A121 (167.6629, 112.2825) -> (167.1745, 112.2904) centre (167.2947, 104.7041) ccw projected
  arc A122 (167.8011, 111.9077) -> (167.6629, 112.2825) centre (148.5, 105) ccw projected
  arc A123 (167.4349, 111.5844) -> (167.8011, 111.9077) centre (162.5994, 117.4312) ccw projected
  arc A124 (167.1234, 111.3425) -> (167.4349, 111.5844) centre (163.3512, 116.5222) ccw projected
  arc A125 (166.8672, 111.1673) -> (167.1234, 111.3425) centre (164.0199, 115.6041) ccw projected
  arc A126 (166.9844, 110.8066) -> (166.8672, 111.1673) centre (148.5, 105) ccw projected
  arc A127 (167.2947, 110.8154) -> (166.9844, 110.8066) centre (167.2888, 105.5434) ccw projected
  arc A128 (167.6889, 110.8028) -> (167.2947, 110.8154) centre (167.2875, 104.4076) ccw projected
  arc A129 (168.1752, 110.7565) -> (167.6889, 110.8028) centre (167.2136, 103.2304) ccw projected
  arc A130 (168.2836, 110.372) -> (168.1752, 110.7565) centre (148.5, 105) ccw projected
  arc A131 (167.8932, 110.0785) -> (168.2836, 110.372) centre (163.5313, 116.2867) ccw projected
  arc A132 (167.5636, 109.8618) -> (167.8932, 110.0785) centre (164.2095, 115.3215) ccw projected
  arc A133 (167.2945, 109.7072) -> (167.5636, 109.8618) centre (164.804, 114.3537) ccw projected
  arc A134 (167.383, 109.3384) -> (167.2945, 109.7072) centre (148.5, 105) ccw projected
  arc A135 (167.693, 109.3228) -> (167.383, 109.3384) centre (167.2735, 104.0676) ccw projected
  arc A136 (168.085, 109.2793) -> (167.693, 109.3228) centre (167.1831, 102.9354) ccw projected
  arc A137 (168.5662, 109.1951) -> (168.085, 109.2793) centre (167.017, 101.7676) ccw projected
  arc A138 (168.6441, 108.8033) -> (168.5662, 109.1951) centre (148.5, 105) ccw projected
  arc A139 (168.2318, 108.5413) -> (168.6441, 108.8033) centre (164.3705, 115.0726) ccw projected
  arc A140 (167.8863, 108.3511) -> (168.2318, 108.5413) centre (164.9708, 114.0571) ccw projected
  arc A141 (167.6059, 108.2181) -> (167.8863, 108.3511) centre (165.4876, 113.0457) ccw projected
  arc A142 (167.6652, 107.8435) -> (167.6059, 108.2181) centre (148.5, 105) ccw projected
  arc A143 (167.973, 107.8036) -> (167.6652, 107.8435) centre (167.1425, 102.5975) ccw projected
  arc A144 (168.3604, 107.7295) -> (167.973, 107.8036) centre (166.9635, 101.4759) ccw projected
  arc A145 (168.8335, 107.6078) -> (168.3604, 107.7295) centre (166.7064, 100.3247) ccw projected
  arc A146 (168.8804, 107.2111) -> (168.8335, 107.6078) centre (148.5, 105) ccw projected
  arc A147 (168.4489, 106.9822) -> (168.8804, 107.2111) centre (165.1119, 113.7963) ccw projected
  arc A148 (168.0895, 106.8197) -> (168.4489, 106.9822) centre (165.6307, 112.7369) ccw projected
  arc A149 (167.7995, 106.7091) -> (168.0895, 106.8197) centre (166.0665, 111.6881) ccw projected
  arc A150 (167.8292, 106.331) -> (167.7995, 106.7091) centre (148.5, 105) ccw projected
  arc A151 (168.133, 106.2671) -> (167.8292, 106.331) centre (166.8965, 101.1423) ccw projected
  arc A152 (168.5133, 106.1629) -> (168.133, 106.2671) centre (166.6301, 100.0382) ccw projected
  arc A153 (168.9754, 106.0044) -> (168.5133, 106.1629) centre (166.2834, 98.9106) ccw projected
  arc A154 (168.9911, 105.6052) -> (168.9754, 106.0044) centre (148.5, 105) ccw projected
  arc A155 (168.5429, 105.4109) -> (168.9911, 105.6052) centre (165.7508, 112.4658) ccw projected
  arc A156 (168.1719, 105.2771) -> (168.5429, 105.4109) centre (166.1849, 111.369) ccw projected
  arc A157 (167.8741, 105.1896) -> (168.1719, 105.2771) centre (166.5371, 110.2892) ccw projected
  arc A158 (167.8741, 104.8104) -> (167.8741, 105.1896) centre (148.5, 105) ccw projected
  arc A159 (168.1719, 104.7229) -> (167.8741, 104.8104) centre (166.5371, 99.7108) ccw projected
  arc A160 (168.5429, 104.5891) -> (168.1719, 104.7229) centre (166.1849, 98.631) ccw projected
  arc A161 (168.9911, 104.3948) -> (168.5429, 104.5891) centre (165.7508, 97.5342) ccw projected
  arc A162 (168.9754, 103.9956) -> (168.9911, 104.3948) centre (148.5, 105) ccw projected
  arc A163 (168.5133, 103.8371) -> (168.9754, 103.9956) centre (166.2834, 111.0894) ccw projected
  arc A164 (168.133, 103.7329) -> (168.5133, 103.8371) centre (166.6301, 109.9618) ccw projected
  arc A165 (167.8292, 103.669) -> (168.133, 103.7329) centre (166.8965, 108.8577) ccw projected
  arc A166 (167.7995, 103.2909) -> (167.8292, 103.669) centre (148.5, 105) ccw projected
  arc A167 (168.0895, 103.1803) -> (167.7995, 103.2909) centre (166.0665, 98.3119) ccw projected
  arc A168 (168.4489, 103.0178) -> (168.0895, 103.1803) centre (165.6307, 97.2631) ccw projected
  arc A169 (168.8804, 102.7889) -> (168.4489, 103.0178) centre (165.1119, 96.2037) ccw projected
  arc A170 (168.8335, 102.3922) -> (168.8804, 102.7889) centre (148.5, 105) ccw projected
  arc A171 (168.3604, 102.2705) -> (168.8335, 102.3922) centre (166.7064, 109.6753) ccw projected
  arc A172 (167.973, 102.1964) -> (168.3604, 102.2705) centre (166.9635, 108.5241) ccw projected
  arc A173 (167.6652, 102.1565) -> (167.973, 102.1964) centre (167.1425, 107.4025) ccw projected
  arc A174 (167.6059, 101.7819) -> (167.6652, 102.1565) centre (148.5, 105) ccw projected
  arc A175 (167.8863, 101.6489) -> (167.6059, 101.7819) centre (165.4876, 96.9543) ccw projected
  arc A176 (168.2318, 101.4587) -> (167.8863, 101.6489) centre (164.9708, 95.9429) ccw projected
  arc A177 (168.6441, 101.1967) -> (168.2318, 101.4587) centre (164.3705, 94.9274) ccw projected
  arc A178 (168.5662, 100.8049) -> (168.6441, 101.1967) centre (148.5, 105) ccw projected
  arc A179 (168.085, 100.7207) -> (168.5662, 100.8049) centre (167.017, 108.2324) ccw projected
  arc A180 (167.693, 100.6772) -> (168.085, 100.7207) centre (167.1831, 107.0646) ccw projected
  arc A181 (167.383, 100.6616) -> (167.693, 100.6772) centre (167.2735, 105.9324) ccw projected
  arc A182 (167.2945, 100.2928) -> (167.383, 100.6616) centre (148.5, 105) ccw projected
  arc A183 (167.5636, 100.1382) -> (167.2945, 100.2928) centre (164.804, 95.6463) ccw projected
  arc A184 (167.8932, 99.9215) -> (167.5636, 100.1382) centre (164.2095, 94.6785) ccw projected
  arc A185 (168.2836, 99.628) -> (167.8932, 99.9215) centre (163.5313, 93.7133) ccw projected
  arc A186 (168.1752, 99.2435) -> (168.2836, 99.628) centre (148.5, 105) ccw projected
  arc A187 (167.6889, 99.1972) -> (168.1752, 99.2435) centre (167.2136, 106.7696) ccw projected
  arc A188 (167.2947, 99.1846) -> (167.6889, 99.1972) centre (167.2875, 105.5924) ccw projected
  arc A189 (166.9844, 99.1934) -> (167.2947, 99.1846) centre (167.2888, 104.4566) ccw projected
  arc A190 (166.8672, 98.8327) -> (166.9844, 99.1934) centre (148.5, 105) ccw projected
  arc A191 (167.1234, 98.6575) -> (166.8672, 98.8327) centre (164.0199, 94.3959) ccw projected
  arc A192 (167.4349, 98.4156) -> (167.1234, 98.6575) centre (163.3512, 93.4778) ccw projected
  arc A193 (167.8011, 98.0923) -> (167.4349, 98.4156) centre (162.5994, 92.5688) ccw projected
  arc A194 (167.6629, 97.7175) -> (167.8011, 98.0923) centre (148.5, 105) ccw projected
  arc A195 (167.1745, 97.7096) -> (167.6629, 97.7175) centre (167.2947, 105.2959) ccw projected
  arc A196 (166.7805, 97.728) -> (167.1745, 97.7096) centre (167.276, 104.1165) ccw projected
  arc A197 (166.4719, 97.7611) -> (166.7805, 97.728) centre (167.1882, 102.9841) ccw projected
  arc A198 (166.3267, 97.4107) -> (166.4719, 97.7611) centre (148.5, 105) ccw projected
  arc A199 (166.5684, 97.2158) -> (166.3267, 97.4107) centre (163.14, 93.2109) ccw projected
  arc A200 (166.86, 96.9503) -> (166.5684, 97.2158) centre (162.4014, 92.3481) ccw projected
  arc A201 (167.1997, 96.5993) -> (166.86, 96.9503) centre (161.5806, 91.5009) ccw projected
  arc A202 (167.0324, 96.2365) -> (167.1997, 96.5993) centre (148.5, 105) ccw projected
  arc A203 (166.5449, 96.2669) -> (167.0324, 96.2365) centre (167.26, 103.8204) ccw projected
  arc A204 (166.1536, 96.3161) -> (166.5449, 96.2669) centre (167.1488, 102.6461) ccw projected
  arc A205 (165.8485, 96.3733) -> (166.1536, 96.3161) centre (166.9724, 101.524) ccw projected
  arc A206 (165.6763, 96.0354) -> (165.8485, 96.3733) centre (148.5, 105) ccw projected
  arc A207 (165.9019, 95.8222) -> (165.6763, 96.0354) centre (162.1699, 92.0986) ccw projected
  arc A208 (166.1718, 95.5346) -> (165.9019, 95.8222) centre (161.3659, 91.2964) ccw projected
  arc A209 (166.4829, 95.158) -> (166.1718, 95.5346) centre (160.4812, 90.5162) ccw projected
  arc A210 (166.2877, 94.8095) -> (166.4829, 95.158) centre (148.5, 105) ccw projected
  arc A211 (165.8041, 94.878) -> (166.2877, 94.8095) centre (167.1096, 102.3522) ccw projected
  arc A212 (165.4178, 94.9578) -> (165.8041, 94.878) centre (166.9067, 101.1901) ccw projected
  arc A213 (165.1182, 95.0388) -> (165.4178, 94.9578) centre (166.6428, 100.0854) ccw projected
  arc A214 (164.92, 94.7154) -> (165.1182, 95.0388) centre (148.5, 105) ccw projected
  arc A215 (165.1282, 94.4852) -> (164.92, 94.7154) centre (161.1156, 91.0659) ccw projected
  arc A216 (165.3747, 94.1773) -> (165.1282, 94.4852) centre (160.2511, 90.3292) ccw projected
  arc A217 (165.6553, 93.7774) -> (165.3747, 94.1773) centre (159.3078, 89.6208) ccw projected
  arc A218 (165.4334, 93.4453) -> (165.6553, 93.7774) centre (148.5, 105) ccw projected
  arc A219 (164.9566, 93.5515) -> (165.4334, 93.4453) centre (166.8445, 100.9002) ccw projected
  arc A220 (164.5778, 93.6614) -> (164.9566, 93.5515) centre (166.551, 99.7577) ccw projected
  arc A221 (164.2854, 93.7656) -> (164.5778, 93.6614) centre (166.2012, 98.6771) ccw projected
  arc A222 (164.0625, 93.4588) -> (164.2854, 93.7656) centre (148.5, 105) ccw projected
  arc A223 (164.252, 93.2129) -> (164.0625, 93.4588) centre (159.9834, 90.119) ccw projected
  arc A224 (164.4735, 92.8866) -> (164.252, 93.2129) centre (159.0638, 89.4524) ccw projected
  arc A225 (164.7219, 92.466) -> (164.4735, 92.8866) centre (158.0679, 88.8202) ccw projected
  arc A226 (164.4746, 92.1523) -> (164.7219, 92.466) centre (148.5, 105) ccw projected
  arc A227 (164.0076, 92.2957) -> (164.4746, 92.1523) centre (166.4663, 99.4736) ccw projected
  arc A228 (163.6386, 92.4349) -> (164.0076, 92.2957) centre (166.0841, 98.3576) ccw projected
  arc A229 (163.3553, 92.5617) -> (163.6386, 92.4349) centre (165.6506, 97.3078) ccw projected
  arc A230 (163.109, 92.2734) -> (163.3553, 92.5617) centre (148.5, 105) ccw projected
  arc A231 (163.2786, 92.0134) -> (163.109, 92.2734) centre (158.7805, 89.2639) ccw projected
  arc A232 (163.4738, 91.6707) -> (163.2786, 92.0134) centre (157.8114, 88.6715) ccw projected
  arc A233 (163.6885, 91.2319) -> (163.4738, 91.6707) centre (156.7689, 88.1194) ccw projected
  arc A234 (163.4173, 90.9386) -> (163.6885, 91.2319) centre (148.5, 105) ccw projected
  arc A235 (162.963, 91.1181) -> (163.4173, 90.9386) centre (165.9773, 98.081) ccw projected
  arc A236 (162.6061, 91.2859) -> (162.963, 91.1181) centre (165.5087, 96.9985) ccw projected
  arc A237 (162.3336, 91.4345) -> (162.6061, 91.2859) centre (164.9942, 95.9859) ccw projected
  arc A238 (162.0655, 91.1664) -> (162.3336, 91.4345) centre (148.5, 105) ccw projected
  arc A239 (162.2141, 90.8939) -> (162.0655, 91.1664) centre (157.5141, 88.5058) ccw projected
  arc A240 (162.3819, 90.537) -> (162.2141, 90.8939) centre (156.5015, 87.9913) ccw projected
  arc A241 (162.5614, 90.0827) -> (162.3819, 90.537) centre (155.419, 87.5227) ccw projected
  arc A242 (162.2681, 89.8115) -> (162.5614, 90.0827) centre (148.5, 105) ccw projected
  arc A243 (161.8293, 90.0261) -> (162.2681, 89.8115) centre (165.3806, 96.7311) ccw projected
  arc A244 (161.4866, 90.2214) -> (161.8293, 90.0261) centre (164.8285, 95.6886) ccw projected
  arc A245 (161.2266, 90.391) -> (161.4866, 90.2214) centre (164.2361, 94.7195) ccw projected
  arc A246 (160.9383, 90.1447) -> (161.2266, 90.391) centre (148.5, 105) ccw projected
  arc A247 (161.0651, 89.8614) -> (160.9383, 90.1447) centre (156.1922, 87.8494) ccw projected
  arc A248 (161.2043, 89.4924) -> (161.0651, 89.8614) centre (155.1424, 87.4159) ccw projected
  arc A249 (161.3477, 89.0254) -> (161.2043, 89.4924) centre (154.0264, 87.0337) ccw projected
  arc A250 (161.034, 88.7781) -> (161.3477, 89.0254) centre (148.5, 105) ccw projected
  arc A251 (160.6134, 89.0265) -> (161.034, 88.7781) centre (164.6798, 95.4321) ccw projected
  arc A252 (160.2871, 89.248) -> (160.6134, 89.0265) centre (164.0476, 94.4362) ccw projected
  arc A253 (160.0412, 89.4375) -> (160.2871, 89.248) centre (163.381, 93.5166) ccw projected
  arc A254 (159.7344, 89.2146) -> (160.0412, 89.4375) centre (148.5, 105) ccw projected
  arc A255 (159.8386, 88.9222) -> (159.7344, 89.2146) centre (154.8229, 87.2988) ccw projected
  arc A256 (159.9485, 88.5434) -> (159.8386, 88.9222) centre (153.7423, 86.949) ccw projected
  arc A257 (160.0547, 88.0666) -> (159.9485, 88.5434) centre (152.5998, 86.6555) ccw projected
  arc A258 (159.7226, 87.8447) -> (160.0547, 88.0666) centre (148.5, 105) ccw projected
  arc A259 (159.3227, 88.1253) -> (159.7226, 87.8447) centre (163.8792, 94.1922) ccw projected
  arc A260 (159.0148, 88.3718) -> (159.3227, 88.1253) centre (163.1708, 93.2489) ccw projected
  arc A261 (158.7846, 88.58) -> (159.0148, 88.3718) centre (162.4341, 92.3844) ccw projected
  arc A262 (158.4612, 88.3818) -> (158.7846, 88.58) centre (148.5, 105) ccw projected
  arc A263 (158.5422, 88.0822) -> (158.4612, 88.3818) centre (153.4146, 86.8572) ccw projected
  arc A264 (158.622, 87.6959) -> (158.5422, 88.0822) centre (152.3099, 86.5933) ccw projected
  arc A265 (158.6905, 87.2123) -> (158.622, 87.6959) centre (151.1478, 86.3904) ccw projected
  arc A266 (158.342, 87.0171) -> (158.6905, 87.2123) centre (148.5, 105) ccw projected
  arc A267 (157.9654, 87.3282) -> (158.342, 87.0171) centre (162.9838, 93.0188) ccw projected
  arc A268 (157.6778, 87.5981) -> (157.9654, 87.3282) centre (162.2036, 92.1341) ccw projected
  arc A269 (157.4646, 87.8237) -> (157.6778, 87.5981) centre (161.4014, 91.3301) ccw projected
  arc A270 (157.1267, 87.6515) -> (157.4646, 87.8237) centre (148.5, 105) ccw projected
  arc A271 (157.1839, 87.3464) -> (157.1267, 87.6515) centre (151.976, 86.5276) ccw projected
  arc A272 (157.2331, 86.9551) -> (157.1839, 87.3464) centre (150.8539, 86.3512) ccw projected
  arc A273 (157.2635, 86.4676) -> (157.2331, 86.9551) centre (149.6796, 86.24) ccw projected
  arc A274 (156.9007, 86.3003) -> (157.2635, 86.4676) centre (148.5, 105) ccw projected
  arc A275 (156.5497, 86.64) -> (156.9007, 86.3003) centre (161.9991, 91.9194) ccw projected
  arc A276 (156.2842, 86.9316) -> (156.5497, 86.64) centre (161.1519, 91.0986) ccw projected
  arc A277 (156.0893, 87.1733) -> (156.2842, 86.9316) centre (160.2891, 90.36) ccw projected
  arc A278 (155.7389, 87.0281) -> (156.0893, 87.1733) centre (148.5, 105) ccw projected
  arc A279 (155.772, 86.7195) -> (155.7389, 87.0281) centre (150.5159, 86.3118) ccw projected
  arc A280 (155.7904, 86.3255) -> (155.772, 86.7195) centre (149.3835, 86.224) ccw projected
  arc A281 (155.7825, 85.8371) -> (155.7904, 86.3255) centre (148.2041, 86.2053) ccw projected
  arc A282 (155.4077, 85.6989) -> (155.7825, 85.8371) centre (148.5, 105) ccw projected
  arc A283 (155.0844, 86.0651) -> (155.4077, 85.6989) centre (160.9312, 90.9006) ccw projected